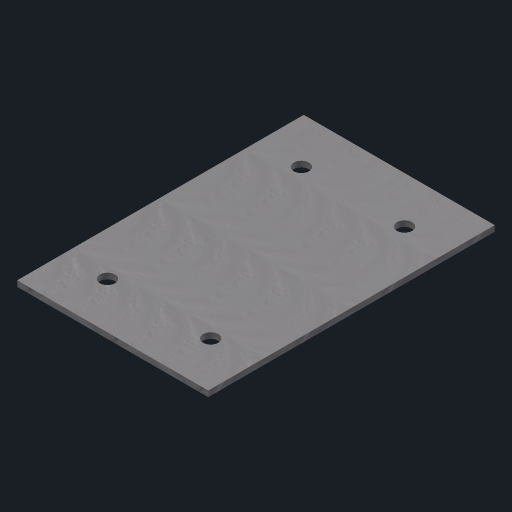
# Autodesk Inventor part: PLACA
Saved by Autodesk Inventor 2024.3 (Build 283343000, 343)
## iProperties
Created: 2024-06-03
Part Number: PLACA
Material: Steel, Mild, Welded
Document SubType Name: Modeling
Designer: Niler
Density: 7.85 g/cm^3
Appearance: Weld - Steel Mild
Author: Niler
Autodesk Inventor part; units mm, degrees
ref_plane "YZ Plane" through (0, 0, 0) normal (1, 0, 0) x (0, 1, 0)
ref_plane "XZ Plane" through (0, 0, 0) normal (0, 1, 0) x (-1, 0, 0)
ref_plane "XY Plane" through (0, 0, 0) normal (0, 0, 1) x (1, 0, 0)
sketch "Sketch1" plane through (0, 0, 0) normal (0, 1, 0) x (-1, 0, 0)
  line L0 (-50, 75) -> (50, 75)
  line L1 (50, 75) -> (50, -75)
  line L2 (50, -75) -> (-50, -75)
  line L3 (-50, -75) -> (-50, 75)
  circle A0 centre (27, 50.75) radius 4
  line L4 (0, 0) -> (28.2437, 0)
  line L5 (28.2437, 0) -> (0, 0)
  circle A1 centre (27, -50.75) radius 4
  line L6 (0, 0) -> (0, 34.6506)
  circle A2 centre (-27, 50.75) radius 4
  circle A3 centre (-27, -50.75) radius 4
  point P0 (50, 0)
  point P1 (0, -75)
  dimension "d0" = 101.5
  dimension "d1" = 8
  dimension "d2" = 54
  dimension "d3" = 100
  dimension "d4" = 150
  constraints: 14 end point, 4 centre point, 3 equal length, 3 symmetric about line, 2 horizontal, 2 midpoint, 1 horizontal alignment, 1 perpendicular, 1 vertical, 1 vertical alignment, 3 other
  measures "d0" distance of A1.centre A0.centre
  measures "d1" diameter of A0
  measures "d2" distance of A2.centre A0.centre
  measures "d3" distance of L1.end L2.end
  measures "d4" distance of L0.end L1.end
extrude "Extrusion1" add sketch "Sketch1" along normal blind 3
body "Solid1"
